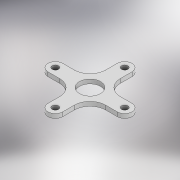
# Autodesk Inventor part: Base Motor
Saved by Autodesk Inventor 2021.4 (Build 254397000, 397)
## iProperties
Created: 2022-12-11
Part Number: Base Motor
Material: Genérico
Document SubType Name: Modeling
Designer: crist
Density: 1 g/cm^3
Appearance: Valor por defecto
Author: crist
Autodesk Inventor part; units mm, degrees
ref_plane "YZ Plane" through (0, 0, 0) normal (1, 0, 0) x (0, 1, 0)
ref_plane "XZ Plane" through (0, 0, 0) normal (0, 1, 0) x (-1, 0, 0)
ref_plane "XY Plane" through (0, 0, 0) normal (0, 0, 1) x (1, 0, 0)
sketch "Boceto1" plane through (0, 0, 0) normal (0, 1, 0) x (-1, 0, 0)
  circle A0 centre (16.5, 0) radius 1.5
  circle A1 centre (0, -16.5) radius 1.5
  circle A2 centre (-16.5, 0) radius 1.5
  circle A3 centre (0, 16.5) radius 1.5
  line L0 (3.5, 11) -> (3.5, 16.5)
  line L1 (3.5, -16.5) -> (3.5, -11)
  line L2 (11, -3.5) -> (16.5, -3.5)
  line L3 (-16.5, -3.5) -> (-11, -3.5)
  arc A4 (3.5, 16.5) -> (-3.5, 16.5) centre (0, 16.5) ccw
  arc A5 (16.5, -3.5) -> (16.5, 3.5) centre (16.5, 0) ccw
  arc A6 (-3.5, -16.5) -> (3.5, -16.5) centre (0, -16.5) ccw
  arc A7 (-16.5, 3.5) -> (-16.5, -3.5) centre (-16.5, 0) ccw
  line L4 (16.5, 3.5) -> (11, 3.5)
  line L5 (-11, 3.5) -> (-16.5, 3.5)
  line L6 (-3.5, 16.5) -> (-3.5, 11)
  line L7 (-3.5, -11) -> (-3.5, -16.5)
  arc A8 (11, -3.5) -> (3.5, -11) centre (11, -11) ccw
  arc A9 (-3.5, -11) -> (-11, -3.5) centre (-11, -11) ccw
  arc A10 (-11, 3.5) -> (-3.5, 11) centre (-11, 11) ccw
  arc A11 (3.5, 11) -> (11, 3.5) centre (11, 11) ccw
  circle A12 centre (0, 0) radius 5
  dimension "d12" = 7.5
  dimension "d15" = 10
  constraints: 16 end point, 16 point on circle, 13 centre point, 12 tangent, 4 coincident, 3 equal radius
  measures "d12" radius of A8
  measures "d15" diameter of A12
extrude "Extrusión1" add sketch "Boceto1" along normal blind 2
